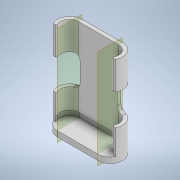
# Autodesk Inventor part: Proto-Valve Holder
Saved by Autodesk Inventor 2020 (Build 240168000, 168)
## iProperties
Created: 2019-12-04
Part Number: Proto-Valve Holder
Material: Generic
Document SubType Name: Modeling
Designer: ball
Density: 1 g/cm^3
Appearance: Default
Author: ball
Autodesk Inventor part; units mm, degrees
ref_plane "YZ Plane" through (0, 0, 0) normal (1, 0, 0) x (0, 1, 0)
ref_plane "XZ Plane" through (0, 0, 0) normal (0, 1, 0) x (-1, 0, 0)
ref_plane "XY Plane" through (0, 0, 0) normal (0, 0, 1) x (1, 0, 0)
sketch "Sketch1" plane through (0, 0, 0) normal (0, 1, 0) x (-1, 0, 0)
  line L0 (-24.3078, -15.4178) -> (21.4122, -15.4178)
  line L1 (21.4122, 12.5222) -> (-24.3078, 12.5222)
  arc A0 (21.4122, -15.4178) -> (21.4122, 12.5222) centre (21.4122, -1.4478) ccw
  arc A1 (-24.3078, 12.5222) -> (-24.3078, -15.4178) centre (-24.3078, -1.4478) ccw
  point P0 (0, 0)
  dimension "d2" = 27.94
  dimension "d3" = 45.72
  constraints: 4 end point, 4 point on circle, 4 tangent, 2 centre point, 1 horizontal, 1 parallel
  measures "d2" distance between parallel lines of L0 L1
  measures "d3" distance of A1.centre A0.centre
extrude "Extrusion1" add sketch "Sketch1" along normal blind 101.6
sketch "Sketch2" plane through (0, 101.6, 0) normal (0, 1, 0) x (1, 0, 0)
  line L0 (24.2727, 11.1519) -> (-21.4473, 11.1519)
  line L1 (-21.4473, -9.1681) -> (24.2727, -9.1681)
  arc A0 (-21.4473, 11.1519) -> (-21.4473, -9.1681) centre (-21.4473, 0.9919) ccw
  arc A1 (24.2727, -9.1681) -> (24.2727, 11.1519) centre (24.2727, 0.9919) ccw
  arc A2 (-21.4122, 15.4178) -> (-21.4122, -12.5222) centre (-21.4122, 1.4478) ccw projected
  point P0 (0, 0)
  dimension "d7" = 20.32
  dimension "d8" = 45.72
  constraints: 4 end point, 4 point on circle, 4 tangent, 2 centre point, 1 horizontal, 1 parallel
  measures "d7" distance between parallel lines of L0 L1
  measures "d8" distance of A1.centre A0.centre
extrude "Extrusion2" cut sketch "Sketch2" against normal blind 95.25
sketch "Sketch3" plane through (0, 6.35, 0) normal (0, 1, 0) x (1, 0, 0)
  arc A0 (-21.4122, 15.4178) -> (-21.4122, -12.5222) centre (-21.4122, 1.4478) ccw projected
  line L0 (-33.8556, -4.9022) -> (40.6958, -4.9022)
  line L1 (40.6958, -4.9022) -> (40.6958, -12.5222)
  line L2 (40.6958, -12.5222) -> (-33.8556, -12.5222)
  line L3 (-33.8556, -12.5222) -> (-33.8556, -4.9022)
  line L4 (-21.4122, -12.5222) -> (24.3078, -12.5222) projected
  point P0 (0, 0)
  dimension "d13" = 7.62
  dimension "d14" = 0
  constraints: 8 end point, 2 parallel, 1 horizontal, 1 perpendicular, 1 point on circle
  measures "d13" distance of L0.end L1.end
  measures "d14" distance between parallel lines of L2 L4
extrude "Extrusion3" cut sketch "Sketch3" along normal blind 95.25
fillet "Fillet1" radius 0.635 3 edges at (32.5483, 53.975, 4.9022) (-29.7228, 53.975, 4.9022) (-33.8556, 53.975, 4.9022)
ref_plane "Work Plane1" through (-21.4473, 101.6, -11.1519) normal (-1, 0, 0) x (0, -1, 0)
ref_plane "Work Plane2" through (24.2727, 101.6, -11.1519) normal (-1, 0, 0) x (0, -1, 0)
sketch "Sketch6" plane through (24.2727, 101.6, -11.1519) normal (-1, 0, 0) x (0, -1, 0)
  line L0 (66.929, 0.4433) -> (32.131, 0.4433)
  line L1 (32.131, 0.4433) -> (32.131, 26.3545)
  line L2 (32.131, 26.3545) -> (66.929, 26.3545)
  line L3 (66.929, 26.3545) -> (66.929, 0.4433)
  line L4 (95.25, 16.0541) -> (95.25, 23.6741) projected
  point P0 (101.6, 11.1519)
  point P1 (95.25, 16.0541)
  dimension "d30" = 34.798
  dimension "d31" = 28.321
  constraints: 8 end point, 2 parallel, 1 horizontal, 1 perpendicular
  measures "d30" distance of L1.end L2.end
  measures "d31" distance between parallel lines of L3 L4
extrude "Extrusion6" cut sketch "Sketch6" against normal up to next
sketch "Sketch7" plane through (-21.4473, 101.6, -11.1519) normal (-1, 0, 0) x (0, -1, 0)
  line L0 (31.75, 1.1631) -> (66.04, 1.1631)
  line L1 (66.04, 1.1631) -> (66.04, 21.3162)
  line L2 (66.04, 21.3162) -> (31.75, 21.3162)
  line L3 (31.75, 21.3162) -> (31.75, 1.1631)
  line L4 (95.25, 15.6913) -> (95.25, 23.6741) projected
  point P0 (101.6, 11.1519)
  dimension "d35" = 34.29
  dimension "d36" = 29.21
  constraints: 8 end point, 2 parallel, 1 horizontal, 1 perpendicular
  measures "d35" distance of L2.end L1.end
  measures "d36" distance between parallel lines of L1 L4
extrude "Extrusion7" cut sketch "Sketch7" along normal blind 25.4
sketch "Sketch10" plane through (-21.4473, 101.6, -11.1519) normal (0, 0, 1) x (1, 0, 0)
  line L0 (-13.9903, -31.75) -> (1.8847, -31.75)
  line L1 (1.8847, -31.75) -> (1.8847, -66.04)
  line L2 (1.8847, -66.04) -> (-13.9903, -66.04)
  line L3 (-13.9903, -66.04) -> (-13.9903, -31.75)
  line L4 (59.7251, -101.6) -> (59.7251, 0) projected
  line L5 (59.7251, -32.131) -> (43.8501, -32.131)
  line L6 (43.8501, -32.131) -> (43.8501, -66.929)
  line L7 (43.8501, -66.929) -> (59.7251, -66.929)
  line L8 (59.7251, -66.929) -> (59.7251, -32.131)
  line L9 (55.1473, -32.131) -> (58.1985, -32.131) projected
  point P0 (21.4473, -101.6)
  dimension "d58" = 15.875
  dimension "d59" = 34.29
  dimension "d60" = 15.875
  dimension "d61" = 34.798
  dimension "d62" = 0
  constraints: 16 end point, 4 parallel, 2 horizontal, 2 perpendicular, 1 point on line
  measures "d58" distance of L1.end L2.end
  measures "d59" distance of L0.end L1.end
  measures "d60" distance of L7.end L6.end
  measures "d61" distance of L6.end L5.end
  measures "d62" distance between parallel lines of L9 L5
extrude "Extrusion10" cut sketch "Sketch10" against normal through all both and the other way through all
fillet "Fillet6" radius 6.35 4 edges at (22.4028, 69.469, -13.2849) (22.4028, 34.671, -13.2849) (-19.5625, 69.85, -13.2849) (-19.5625, 35.56, -13.2849)
sketch "Sketch11" plane through (0, 6.35, 0) normal (0, 1, 0) x (1, 0, 0)
  arc A0 (33.1455, -3.9578) -> (24.2727, 11.1519) centre (24.2727, 0.9919) ccw projected
  arc A1 (24.2727, -10.5778) -> (24.2727, 12.5616) centre (24.2727, 0.9919) ccw
  arc A2 (-21.4473, 11.1519) -> (-30.32, -3.9578) centre (-21.4473, 0.9919) ccw projected
  arc A3 (-21.4473, 12.5616) -> (-20.3359, -10.5243) centre (-21.4473, 0.9919) ccw
  line L0 (24.2727, 12.5616) -> (-24.2727, 12.5616)
  line L1 (-20.4393, -10.5778) -> (24.2727, 12.5616) construction
  line L2 (20.4393, -10.5778) -> (-24.2727, 12.5616) construction
  line L3 (24.2727, -10.5778) -> (-21.4473, -10.5778)
  line L4 (-24.2727, 12.5616) -> (-24.2727, 10.7512)
  line L5 (24.2727, 0.9919) -> (24.2727, 12.5616)
  point P0 (0, 0)
  dimension "d66" = 23.1394
  dimension "d67" = 23.1394
  constraints: 12 end point, 6 point on circle, 6 point on line, 2 centre point, 2 coincident, 1 parallel, 1 tangent
  measures "d66" diameter of A1
  measures "d67" diameter of A3
extrude "Extrusion11" cut sketch "Sketch11" along normal blind 6.35 contours L3 A3 L0 A1
body "Solid1"
